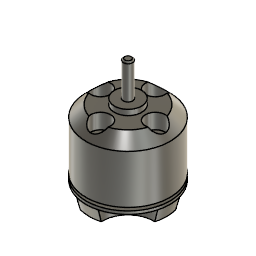
brushless-motor (Autodesk Fusion 360 design; units mm, degrees)
part number: 2026-06-20-16-16-47-686
Autodesk Fusion 360 part; units mm, degrees
sketch "Sketch1" plane through (0, 0, 0) normal (0, 0, 1) x (1, 0, 0)
  circle A0 centre (0, 0) radius 138.5
  line L0 (0, 138.5) -> (0, -138.5) construction
  line L1 (0, 0) -> (138.5, 0) construction
  line L2 (0, 0) -> (-138.5, 0) construction
  arc A1 (36, 133.7395) -> (133.7395, 36) centre (118.6299, 118.6299) ccw
  arc A2 (-133.7395, 36) -> (-36, 133.7395) centre (-118.6299, 118.6299) ccw
  arc A3 (-36, -133.7395) -> (-133.7395, -36) centre (-118.6299, -118.6299) ccw
  arc A4 (133.7395, -36) -> (36, -133.7395) centre (118.6299, -118.6299) ccw
  dimension "d1" = 277
  dimension "d2" = 277
  dimension "d3" = 277
  dimension "d4" = 84
  dimension "d5" = 36
  dimension "d6" = 36
  constraint coincident A0.centre L1.start
  constraint coincident A0 L0.start
  constraint coincident A0 L0.end
  constraint vertical L0
  constraint coincident A0 L1.end
  constraint perpendicular L0 L1
  constraint coincident A0 L2.end
  constraint perpendicular L0 L2
  constraint coincident A0 A1.end
  constraint coincident A0 A1.start
  constraint symmetric L0 A1.start A2.end
  constraint symmetric L0 A1.end A2.start
  constraint symmetric L0 A1 A2
  constraint symmetric L2 A1.start A4.end
  constraint symmetric L2 A1.end A4.start
  constraint symmetric L2 A1 A4
  constraint symmetric L2 A2.end A3.start
  constraint symmetric L2 A2.start A3.end
  constraint symmetric L2 A2 A3
  measures "d1" diameter of A0
  measures "d2" distance of L0.start L0.end
  measures "d3" distance of L1.end L2.end
  measures "d4" radius of A1
  measures "d5" horizontal distance of A0.centre A1.start
  measures "d6" vertical distance of A0.centre A1.end
extrude "Extrude1" add sketch "Sketch1" along normal blind 40 contours A0 A1 A2 A3 A4
draft "Draft1" angle -15 neutral plane through (0, 0, 0) pull (0, 0, -1) 4 faces at (-24.1547, -136.3774, 13.3333) (135.1883, -30.1062, 26.6667) (-30.1062, 135.1883, 13.3333) (-136.3774, -24.1547, 26.6667)
sketch "Sketch4" plane through (0, 0, 40) normal (0, 0, 1) x (-1, 0, 0)
  arc A0 (-34.742, -122.9685) -> (34.742, -122.9685) centre (0, 0) ccw
  arc A1 (122.9685, -34.742) -> (34.742, -122.9685) centre (118.6299, -118.6299) ccw
  arc A2 (122.9685, -34.742) -> (122.9685, 34.742) centre (0, 0) ccw
  arc A3 (34.742, 122.9685) -> (122.9685, 34.742) centre (118.6299, 118.6299) ccw
  arc A4 (34.742, 122.9685) -> (-34.742, 122.9685) centre (0, 0) ccw
  arc A5 (-122.9685, 34.742) -> (-34.742, 122.9685) centre (-118.6299, 118.6299) ccw
  arc A6 (-122.9685, 34.742) -> (-122.9685, -34.742) centre (0, 0) ccw
  arc A7 (-34.742, -122.9685) -> (-122.9685, -34.742) centre (-118.6299, -118.6299) ccw
  circle A8 centre (0, 0) radius 15.5
  dimension "d14" = 31
  constraint coincident A0.centre A2.centre
  measures "d14" diameter of A8
extrude "Extrude2" add sketch "Sketch4" along normal blind 10 contours A8
sketch "Sketch5" plane through (0, 0, 40) normal (0, 0, 1) x (-1, 0, 0)
  circle A0 centre (0, 0) radius 15.5
  arc A1 (-34.742, -122.9685) -> (34.742, -122.9685) centre (0, 0) ccw
  arc A2 (122.9685, -34.742) -> (34.742, -122.9685) centre (118.6299, -118.6299) ccw
  arc A3 (122.9685, -34.742) -> (122.9685, 34.742) centre (0, 0) ccw
  arc A4 (34.742, 122.9685) -> (122.9685, 34.742) centre (118.6299, 118.6299) ccw
  arc A5 (34.742, 122.9685) -> (-34.742, 122.9685) centre (0, 0) ccw
  arc A6 (-122.9685, 34.742) -> (-34.742, 122.9685) centre (-118.6299, 118.6299) ccw
  arc A7 (-122.9685, 34.742) -> (-122.9685, -34.742) centre (0, 0) ccw
  arc A8 (-34.742, -122.9685) -> (-122.9685, -34.742) centre (-118.6299, -118.6299) ccw
  circle A9 centre (0, 100) radius 9.5
  line L0 (-127.782, 0) -> (127.782, 0) construction
  line L1 (0, 127.782) -> (0, -127.782) construction
  circle A10 centre (0, -100) radius 9.5
  line L2 (0, 0) -> (100, 100) construction
  circle A11 centre (100, 0) radius 9.5
  circle A12 centre (-100, 0) radius 9.5
  dimension "d17" = 19
  dimension "d19" = 100
  constraint midpoint A7 L0.start
  constraint midpoint A3 L0.end
  constraint midpoint A5 L1.start
  constraint midpoint A1 L1.end
  constraint symmetric A9 L0 A10
  constraint coincident A0.centre A1.centre
  constraint symmetric A9 L2 A11
  constraint symmetric L1 A11 A12
  measures "d17" diameter of A9
  measures "d19" distance of A0.centre A9.centre
extrude "Extrude3" cut sketch "Sketch5" against normal up to surface (40 mm away) contours A9 | A10 | A11 | A12
sketch "Sketch6" plane through (0, 0, 0) normal (0, 0, -1) x (1, 0, 0)
  circle A0 centre (-100, 0) radius 9.5
  circle A1 centre (100, 0) radius 9.5
  circle A2 centre (0, 100) radius 9.5
  circle A3 centre (0, -100) radius 9.5
  arc A4 (-36, -133.7395) -> (36, -133.7395) centre (0, 0) ccw
  arc A5 (133.7395, -36) -> (36, -133.7395) centre (118.6299, -118.6299) ccw
  arc A6 (133.7395, -36) -> (133.7395, 36) centre (0, 0) ccw
  arc A7 (36, 133.7395) -> (133.7395, 36) centre (118.6299, 118.6299) ccw
  arc A8 (36, 133.7395) -> (-36, 133.7395) centre (0, 0) ccw
  arc A9 (-133.7395, 36) -> (-36, 133.7395) centre (-118.6299, 118.6299) ccw
  arc A10 (-133.7395, 36) -> (-133.7395, -36) centre (0, 0) ccw
  arc A11 (-36, -133.7395) -> (-133.7395, -36) centre (-118.6299, -118.6299) ccw
  circle A12 centre (0, 0) radius 138.5
  constraint concentric A4 A12
extrude "Extrude4" add sketch "Sketch6" along normal blind 10 contours A0 | A1 | A2 | A3 | A4 A5 A6 A7 A8 A9 A10 A11 A12 | A11 A12 | A5 A12 | A9 A12 | A7 A12
sketch "Sketch7" plane through (0, 0, -10) normal (0, 0, -1) x (1, 0, 0)
  circle A0 centre (0, 0) radius 138.5
  circle A1 centre (0, 0) radius 118.5
  dimension "d24" = 237
  constraint coincident A0.centre A1.centre
  measures "d24" diameter of A1
extrude "Extrude5" add sketch "Sketch7" along normal blind 10 contours A1
sketch "Sketch8" plane through (0, 0, -20) normal (0, 0, -1) x (1, 0, 0)
  circle A0 centre (0, 0) radius 118.5
  circle A1 centre (0, 0) radius 138.5
  dimension "d27" = 277
  constraint coincident A0.centre A1.centre
  measures "d27" diameter of A1
extrude "Extrude6" add sketch "Sketch8" along normal blind 196 contours A0 | A1
chamfer "Chamfer2" distance 36 angle 45 1 edges at (-129.1273, 50.0837, -216)
sketch "Sketch9" plane through (0, 0, -216) normal (0, 0, -1) x (1, 0, 0)
  circle A0 centre (0, 0) radius 102.5
  circle A1 centre (0, 0) radius 45
  dimension "d31" = 90
  constraint coincident A0.centre A1.centre
  measures "d31" diameter of A1
extrude "Extrude7" add sketch "Sketch9" along normal blind 18 contours A1
sketch "Sketch10" plane through (0, 0, -234) normal (0, 0, -1) x (1, 0, 0)
  circle A0 centre (0, 0) radius 45
  circle A1 centre (0, 0) radius 15.5
  dimension "d34" = 31
  constraint coincident A0.centre A1.centre
  measures "d34" diameter of A1
extrude "Extrude8" add sketch "Sketch10" along normal blind 114 contours A1
fillet "Fillet2" radius 5 1 edges at (-14.4511, 5.605, -348)
sketch "Sketch11" plane through (0, 0, -216) normal (0, 0, -1) x (1, 0, 0)
  circle A0 centre (0, 0) radius 45
  circle A1 centre (0, 0) radius 102.5
  circle A2 centre (90, 0) radius 32.5
  line L0 (0, 140) -> (0, -140) construction
  line L1 (-140, 0) -> (140, 0) construction
  line L2 (0, 0) -> (150, 150) construction
  circle A3 centre (-90, 0) radius 32.5
  circle A4 centre (0, 90) radius 32.5
  circle A5 centre (0, -90) radius 32.5
  dimension "d39" = 65
  constraint vertical L0
  constraint horizontal L1
  constraint coincident A0.centre A1.centre
  constraint symmetric A2 L0 A3
  constraint symmetric A2 L2 A4
  constraint symmetric L1 A4 A5
  measures "d39" diameter of A2
extrude "Extrude9" cut sketch "Sketch11" against normal blind 50 contours A1 A2 | A1 A2 | A1 A4 | A1 A4 | A1 A5 | A1 A5 | A1 A3 | A1 A3
thread "Thread1" "ISO Metric profile 18.0 M18x2.5 M18x2.5 6H" major diameter 18.2926 minor diameter 15.5187 pitch 2.5 angle 60 resizes the face on face at (-109.4882, 0.4735, 13.3333) on face at (-9.4882, 100.4735, 13.3333) on face at (90.5118, 0.4735, 13.3333) on face at (-9.4882, -99.5265, 13.3333)
move_body "Move1" bodies 1 to x (1, 0, 0) y (0, -1, 0) z (0, 0, -1) at (0, 0, -200)
move_body "Move2" bodies 1 to x (1, 0, 0) y (0, 1, 0) z (0, 0, 1) at (0, 0, 250)
scale "Scale1" factor 0.5 about (-45, 0, 266) bodies 1
equation "d39 = ( 32.5 * 2 ) * 1 mm"
